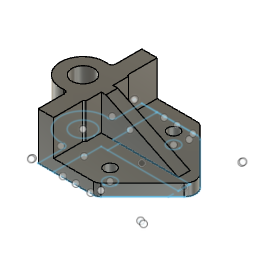
A3 (Autodesk Fusion 360 design; units mm, degrees)
Autodesk Fusion 360 part; units mm, degrees
sketch "Sketch1" plane through (0, 0, 0) normal (0, 0, 1) x (1, 0, 0)
  circle A0 centre (-50, 0) radius 9.5
  arc A1 (-29.5, -18) -> (-31, -19.5) centre (-29.5, -19.5) ccw
  arc A2 (-31, 19.5) -> (-29.5, 18) centre (-29.5, 19.5) ccw
  line L0 (-31, 43) -> (-31, 19.5)
  line L1 (-31, -19.5) -> (-31, -43)
  line L2 (-24, 5) -> (-24, -5)
  line L3 (-50, 43) -> (-50, 44)
  line L4 (-44, 44) -> (2.7447, 44)
  line L5 (42, 44) -> (42, 43)
  line L6 (-50, -43) -> (-50, -44)
  line L7 (-31, -43) -> (-31, -44)
  line L8 (-24, -43) -> (-24, -44)
  line L9 (-13, -43) -> (-13, -44)
  line L10 (42, -43) -> (42, -44)
  line L11 (-13, 43) -> (-13, 44)
  line L12 (-24, 43) -> (-24, 44)
  line L13 (-31, 43) -> (-31, 44)
  line L14 (-31, 44) -> (-44, 44)
  arc A3 (-47.4091, 18.8225) -> (-47.4091, -18.8225) centre (-50, 0) ccw
  line L15 (-44, 44) -> (-44, 21.7945)
  line L16 (-44, -21.7945) -> (-44, -44)
  arc A4 (-47.4091, 18.8225) -> (-44, 21.7945) centre (-47, 21.7945) ccw
  arc A5 (-44, -21.7945) -> (-47.4091, -18.8225) centre (-47, -21.7945) ccw
  line L17 (-31, 44) -> (0, 44)
  line L18 (0, 44) -> (0, 43.393)
  circle A6 centre (0, 27) radius 5
  circle A7 centre (0, -27) radius 5
  line L19 (0, 44) -> (2.7426, 44)
  line L20 (36, 0) -> (36, 5)
  line L21 (36, 5) -> (-29.5, 5)
  line L22 (36, 5) -> (36, -5)
  line L23 (36, -5) -> (-29.5, -5)
  line L24 (45.5, -44) -> (42, -44)
  line L25 (42.7175, -6.7175) -> (7.3388, -42.0962)
  arc A8 (2.7426, -44) -> (7.3388, -42.0962) centre (2.7426, -37.5) ccw
  arc A9 (0, -31.607) -> (-0.6526, -31.9572) centre (2.7426, -37.5) ccw
  line L26 (0, -44) -> (0, -43.393)
  line L27 (0, -32) -> (0, -31.607)
  line L28 (-44, -44) -> (2.7426, -44)
  line L29 (42.7175, 6.7175) -> (7.3388, 42.0962)
  arc A10 (7.3388, 42.0962) -> (2.7406, 44) centre (2.7426, 37.5) ccw
  arc A11 (42.7175, -6.7175) -> (42.7175, 6.7175) centre (36, 0) ccw
  line L30 (36, 5) -> (36, -5)
  line L31 (36, -9.5) -> (36, -13.435)
  line L32 (-29.5, 18) -> (-29.5, 5)
  line L33 (-29.5, -5) -> (-29.5, -18)
  dimension "d10" = 19
  dimension "d11" = 19
  dimension "d18" = 3
  dimension "d19" = 3
  dimension "d22" = 92
  dimension "d25" = 88
  dimension "d26" = 13
  dimension "d28" = 6
  dimension "d29" = 6
  dimension "d30" = 20
  dimension "d31" = 31
  dimension "d32" = 17
  dimension "d33" = 17
  dimension "d34" = 10
  dimension "d35" = 10
  dimension "d38" = 19
  dimension "d43" = 13
  dimension "d47" = 13
  constraint tangent A2 L0
  constraint tangent A1 L0
  constraint coincident A1.end L0
  constraint collinear L0 L1
  constraint vertical L32
  constraint vertical L3
  constraint perpendicular L3 L4
  constraint perpendicular L6 L28
  constraint coincident L7.end L28
  constraint perpendicular L7 L28
  constraint coincident L8.end L28
  constraint perpendicular L8 L28
  constraint coincident L9.end L28
  constraint perpendicular L9 L28
  constraint perpendicular L10 L28
  constraint coincident L4 L11.end
  constraint perpendicular L4 L11
  constraint coincident L4 L12.end
  constraint perpendicular L4 L12
  constraint coincident L4 L13.end
  constraint perpendicular L4 L13
  constraint perpendicular L13 L14
  constraint perpendicular L15 L28
  constraint concentric A0 A3
  constraint tangent L16 A5
  constraint tangent L15 A4
  constraint tangent A3 A4
  constraint tangent A3 A5
  constraint perpendicular L16 L28
  constraint perpendicular L13 L17
  constraint coincident L26.start L28
  constraint perpendicular L4 L18
  constraint perpendicular L26 L28
  constraint perpendicular L18 L19
  constraint perpendicular L28 L30
  constraint perpendicular L21 L32
  constraint perpendicular L21 L22
  constraint coincident L23.end L32
  constraint perpendicular L23 L32
  constraint coincident L21 L2.start
  constraint coincident L23 L2.end
  constraint coincident L20.start A11.centre
  constraint tangent L25 A11
  constraint coincident L20.start L30
  constraint tangent L25 A8
  constraint tangent A8 L28
  constraint coincident A7 A9.end
  constraint concentric A8 A9
  constraint coincident A7 L27.start
  constraint collinear L26 L27
  constraint coincident L25 L31.end
  constraint tangent L29 A11
  constraint tangent L29 A10
  constraint tangent L19 A10
  constraint coincident A10 L19.end
  constraint coincident A10 L4.end
  constraint coincident L4 A10.end
  constraint coincident L31.start L30
  constraint collinear L30 L31
  constraint collinear L32 L33
  measures "d10" distance of L0.start L3.start
  measures "d11" diameter of A0
  measures "d18" diameter of A1
  measures "d19" diameter of A2
  measures "d22" distance of L3.end L5.start
  measures "d25" distance of L5.start L10.end
  measures "d26" distance of L13.end L4.start
  measures "d28" diameter of A4
  measures "d29" diameter of A5
  measures "d30" distance of L12.end L4.start
  measures "d31" distance of L13.end L17.end
  measures "d32" distance of L17.end A6.centre
  measures "d33" distance of L26.start A7.centre
  measures "d34" diameter of A6
  measures "d35" diameter of A7
  measures "d38" diameter of A11
  measures "d43" diameter of A8
  measures "d47" diameter of A10
extrude "Extrude5" add sketch "Sketch1" along normal blind 40 contours A1 A2 L0 L1 L2 L4 L7 L13 L14 A3 L15 L16 A4 A5 L21 L23 L28 L32 L33
extrude "Extrude6" add sketch "Sketch1" along normal blind 10 contours A1 A2 L0 L1 L4 L7 L13 L17 L19 L20 L21 L22 L23 L25 A8 L28 L29 A10 A11 L30 L32 L33
extrude "Extrude7" add sketch "Sketch1" along normal blind 40 contours L2 L20 L21 L22 L23 L30
sketch "Sketch3" plane through (0, -5, 0) normal (0, -1, 0) x (1, 0, 0)
  line L0 (-29.5, 10) -> (36, 10)
  line L1 (36, 10) -> (36, 40)
  line L2 (36, 40) -> (-29.5, 40)
  line L3 (-29.5, 40) -> (-29.5, 10)
  line L4 (-29.5, 40) -> (-25.5, 40)
  line L5 (-25.5, 40) -> (36, 10)
  dimension "d62" = 4
  constraint coincident L2.end L3.start
  constraint perpendicular L3 L4
  constraint coincident L0.end L1.start
  measures "d62" distance of L2.end L4.end
extrude "Extrude8" cut sketch "Sketch3" against normal blind 10 contours L1 L2 L5
extrude "Extrude2" [suppressed]
extrude "Extrude1" [suppressed]
extrude "Extrude3" [suppressed]
sketch "Sketch2" plane through (0, -5, 0) normal (0, -1, 0) x (1, 0, 0)
  line L0 (-29.5, 10) -> (36, 10)
  line L1 (36, 10) -> (36, 40)
  line L2 (36, 40) -> (-29.5, 40)
  line L3 (-29.5, 40) -> (-29.5, 10)
  line L4 (-29.5, 40) -> (36, 10)
  constraint coincident L2.end L3.start
  constraint coincident L0.end L1.start
extrude "Extrude4" [suppressed]
